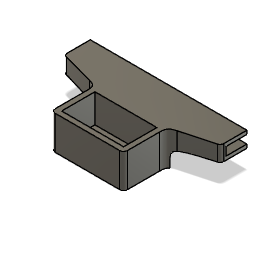
Button Mount (Autodesk Fusion 360 design; units mm, degrees)
Autodesk Fusion 360 part; units mm, degrees
sketch "Sketch1" plane through (0, 0, 0) normal (0, 1, 0) x (1, 0, 0)
  line L0 (0, 0) -> (11.5, 0)
  line L1 (11.5, 0) -> (11.5, 6)
  line L2 (11.5, 6) -> (0, 6)
  line L3 (0, 6) -> (0, 0)
  line L4 (-0.2, -0.2) -> (11.7, -0.2)
  line L5 (11.7, -0.2) -> (11.7, 6.2)
  line L6 (11.7, 6.2) -> (-0.2, 6.2)
  line L7 (-0.2, 6.2) -> (-0.2, -0.2)
  dimension "d1" = 11.5
  dimension "d2" = 6
  dimension "d3" = 0.2
  constraint horizontal L0
  constraint vertical L1
  constraint horizontal L2
  constraint vertical L3
  constraint coincident L0.start L3.end
  measures "d1" distance of L0.start L0.end
  measures "d2" distance of L0.start L2.end
extrude "Extrude1" add sketch "Sketch1" along normal blind 1 contours L0 L1 L2 L3 | L4 L5 L6 L7
sketch "Sketch2" plane through (0, 1, 0) normal (0, 1, 0) x (-1, 0, 0)
  line L0 (0.2, -6.2) -> (0.2, 0.2)
  line L1 (0.2, 0.2) -> (-11.7, 0.2)
  line L2 (-11.7, 0.2) -> (-11.7, -6.2)
  line L3 (-11.7, -6.2) -> (0.2, -6.2)
  line L4 (0.2, 0.2) -> (-11.7, 0.2)
  line L5 (-11.7, 0.2) -> (-11.7, -6.2)
  line L6 (-11.7, -6.2) -> (0.2, -6.2)
  line L7 (0.2, -6.2) -> (0.2, 0.2)
  line L8 (-1.3, -1.3) -> (-10.2, -1.3)
  line L9 (-10.2, -1.3) -> (-10.2, -4.7)
  line L10 (-10.2, -4.7) -> (-1.3, -4.7)
  line L11 (-1.3, -4.7) -> (-1.3, -1.3)
  dimension "d6" = -1.5
  constraint horizontal L4
  constraint vertical L5
  constraint horizontal L6
  constraint vertical L7
  constraint coincident L2.end L3.start
  constraint coincident L0.end L1.start
extrude "Extrude2" cut sketch "Sketch2" against normal blind 1 contours L8 L9 L10 L11
sketch "Sketch3" plane through (0, 0, 0) normal (0, -1, 0) x (1, 0, 0)
  line L0 (1.3, -1.3) -> (10.2, -1.3)
  line L1 (10.2, -1.3) -> (10.2, -4.7)
  line L2 (10.2, -4.7) -> (1.3, -4.7)
  line L3 (1.3, -4.7) -> (1.3, -1.3)
  line L4 (-0.2, 0.2) -> (-0.2, -6.2)
  line L5 (-0.2, -6.2) -> (11.7, -6.2)
  line L6 (11.7, -6.2) -> (11.7, 0.2)
  line L7 (11.7, 0.2) -> (-0.2, 0.2)
  line L8 (-0.2, -6.2) -> (11.7, -6.2)
  line L9 (11.7, -6.2) -> (11.7, 0.2)
  line L10 (11.7, 0.2) -> (-0.2, 0.2)
  line L11 (-0.2, 0.2) -> (-0.2, -6.2)
  line L12 (-1.2, -7.2) -> (12.7, -7.2)
  line L13 (12.7, -7.2) -> (12.7, 1.2)
  line L14 (12.7, 1.2) -> (-1.2, 1.2)
  line L15 (-1.2, 1.2) -> (-1.2, -7.2)
  dimension "d9" = 1
  constraint horizontal L8
  constraint vertical L9
  constraint horizontal L10
  constraint vertical L11
  constraint coincident L6.end L7.start
  constraint coincident L4.end L5.start
extrude "Extrude3" add sketch "Sketch3" against normal blind 7 contours L12 L13 L14 L15
ref_plane "WorkPlane1" through (5.75, 3.5, -3) normal (0, 1, 0) x (0, 0, 1)
sketch "Sketch4" plane through (5.75, 3.5, -3) normal (0, 1, 0) x (1, 0, 0)
  circle A0 centre (0, 56.7) radius 52.5
  line L0 (6.95, 4.2) -> (15.0371, 6.3996)
  line L1 (15.0371, 6.3996) -> (-15.0371, 6.3996)
  line L2 (-15.0371, 6.3996) -> (-6.95, 4.2)
  line L3 (-6.95, 4.2) -> (6.95, 4.2)
  dimension "d12" = 105
  constraint coincident A0 L0.end
  constraint coincident A0 L1.end
  constraint horizontal L1
  measures "d12" diameter of A0
extrude "Extrude4" add sketch "Sketch4" along normal blind 3 contours A0 L0 L1 L2 | A0 L2 L3 | A0 L0 L3
extrude "Extrude5" add 1 faces at (10.7624, 5.5, -9.3996) along direction (0, 0, -1) blind 5
sketch "Sketch5" plane through (0, 0, -14.3996) normal (0, 0, -1) x (-1, 0, 0)
  line L0 (-20.7871, 3.5) -> (9.2871, 3.5)
  line L1 (9.2871, 3.5) -> (9.2871, 6.5)
  line L2 (9.2871, 6.5) -> (-20.7871, 6.5)
  line L3 (-20.7871, 6.5) -> (-20.7871, 3.5)
  line L4 (41.7871, 4.2) -> (-23.2129, 4.2)
  line L5 (-23.2129, 4.2) -> (-23.2129, 5.8)
  line L6 (-23.2129, 5.8) -> (41.7871, 5.8)
  line L7 (41.7871, 5.8) -> (41.7871, 4.2)
  line L8 (41.7871, 4.2) -> (-23.2129, 5.8) construction
  line L9 (-23.2129, 4.2) -> (41.7871, 5.8) construction
  point P0 (9.2871, 5)
  dimension "d17" = 65
  dimension "d18" = 1.6
  constraint horizontal L4
  constraint perpendicular L4 L5
  constraint parallel L4 L6
  constraint parallel L5 L7
  constraint coincident L8 P0
  constraint coincident L9 P0
  constraint midpoint L1 P0
  measures "d17" distance of L5.end L6.end
  measures "d18" distance of L4.end L5.end
extrude "Extrude6" cut sketch "Sketch5" against normal blind 4 contours L1 L3 L4 L6
sketch "Sketch6" plane through (0, 4.2, 0) normal (0, 1, 0) x (-1, 0, 0)
  line L0 (-20.7871, -14.3996) -> (9.2871, -14.3996)
  line L1 (9.2871, -14.3996) -> (9.2871, -10.3996)
  line L2 (9.2871, -10.3996) -> (-20.7871, -10.3996)
  line L3 (-20.7871, -10.3996) -> (-20.7871, -14.3996)
  circle A0 centre (-5.75, -44.1348) radius 36.9349
  constraint coincident L2.end A0
  constraint coincident L1.end A0
extrude "Extrude7" cut sketch "Sketch6" along normal blind 1.6
extrude "Extrude8" cut 1 faces at (3.7667, 7, 0.8667) along direction (0, -1, 0) up to surface (0.5 mm away)
fillet "Fillet2" radius 2 tangency weight 2 3 edges at (12.7, 5, -7.2) (5.75, 3.5, -7.2) (-1.2, 5, -7.2)
fillet "Fillet3" radius 0.75 4 edges at (12.7, 3.25, 1.2) (-1.2, 3.25, 1.2) (-9.2871, 5, -9.3996) (20.7871, 5, -9.3996)
